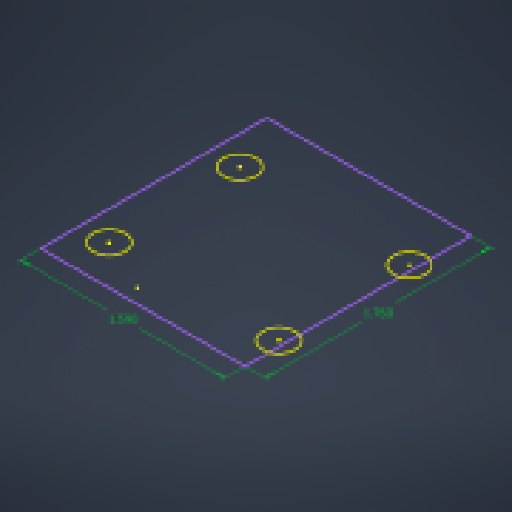
# Autodesk Inventor part: WheelBracketConnector
Saved by Autodesk Inventor 2027 (Build 310192000, 192)
## iProperties
Created: 2026-07-09
Part Number: WheelBracketConnector
Material: Generic
Document SubType Name: Modeling
Designer: belcz
Density: 1 g/cm^3
Appearance: Default
Author: belcz
Autodesk Inventor part; units mm, degrees
ref_plane "YZ Plane" through (0, 0, 0) normal (1, 0, 0) x (0, 1, 0)
ref_plane "XZ Plane" through (0, 0, 0) normal (0, 1, 0) x (-1, 0, 0)
ref_plane "XY Plane" through (0, 0, 0) normal (0, 0, 1) x (1, 0, 0)
sketch "Sketch1" plane through (0, 0, 0) normal (0, 1, 0) x (-1, 0, 0)
  circle A0 centre (10.7243, -30.9952) radius 3.175 projected
  circle A1 centre (10.7243, -5.1761) radius 3.175 projected
  circle A2 centre (-22.8037, -5.1761) radius 3.175 projected
  circle A3 centre (-22.8037, -30.9952) radius 3.175 projected
  line L0 (16.4239, -38.285) -> (-28.2801, -38.285)
  line L1 (-28.2801, -38.285) -> (-28.2801, 2.101)
  line L2 (-28.2801, 2.101) -> (16.4239, 2.101)
  line L3 (16.4239, 2.101) -> (16.4239, -38.285)
  circle A4 centre (-22.8037, -30.9952) radius 3.683
  circle A5 centre (-22.8037, -5.1761) radius 3.683
  circle A6 centre (10.7243, -5.1761) radius 3.683
  circle A7 centre (10.7243, -30.9952) radius 3.683
  line L4 (-28.2801, 2.101) -> (16.4239, 2.101)
  line L5 (16.4239, 2.101) -> (16.4239, -38.285)
  line L6 (16.4239, -38.285) -> (-28.2801, -38.285)
  line L7 (-28.2801, -38.285) -> (-28.2801, 2.101)
  circle A8 centre (10.7243, -5.1761) radius 3.175
  circle A9 centre (10.7243, -30.9952) radius 3.175
  circle A10 centre (-22.8037, -30.9952) radius 3.175
  circle A11 centre (-22.8037, -5.1761) radius 3.175
  point P0 (0, 0)
  dimension "d0" = 44.704
  dimension "d1" = 40.386
  dimension "d2" = 7.2898
  dimension "d3" = 7.2771
  dimension "d4" = 7.366
  dimension "d5" = 7.366
  dimension "d6" = 7.366
  dimension "d7" = 7.366
  constraints: 16 end point, 8 centre point, 8 coincident, 4 concentric, 4 parallel, 2 horizontal, 2 perpendicular
  measures "d0" distance of L1.end L2.end
  measures "d1" distance of L0.end L1.end
  measures "d2" distance from line of L0 A3.centre
  measures "d3" distance from line of L2 A2.centre
  measures "d4" diameter of A4
  measures "d5" diameter of A5
  measures "d6" diameter of A6
  measures "d7" diameter of A7
extrude "Extrusion1" add sketch "Sketch1" along normal blind 4.826 contours A4 | A5 | A6 | A7
sketch "Sketch2" plane through (-10.7243, 0, -30.9952) normal (0, -1, 0) x (1, 0, 0)
  line L0 (39.0044, 33.0962) -> (-5.6996, 33.0962) projected
  line L1 (39.0044, -7.2898) -> (39.0044, 33.0962) projected
  line L2 (-5.6996, -7.2898) -> (39.0044, -7.2898) projected
  line L3 (-5.6996, 33.0962) -> (-5.6996, -7.2898) projected
  line L4 (39.0044, 33.0962) -> (-5.6996, 33.0962)
  line L5 (-5.6996, 33.0962) -> (-5.6996, -7.2898)
  line L6 (-5.6996, -7.2898) -> (39.0044, -7.2898)
  line L7 (39.0044, -7.2898) -> (39.0044, 33.0962)
  circle A0 centre (33.528, 0) radius 3.175 projected
  circle A1 centre (0, 0) radius 3.175 projected
  circle A2 centre (0, 25.8191) radius 3.175 projected
  circle A3 centre (33.528, 25.8191) radius 3.175 projected
  circle A4 centre (33.528, 0) radius 3.175
  circle A5 centre (0, 0) radius 3.175
  circle A6 centre (0, 25.8191) radius 3.175
  circle A7 centre (33.528, 25.8191) radius 3.175
  point P0 (10.7243, 30.9952)
  constraints: 8 end point, 4 centre point, 4 coincident, 4 concentric, 2 parallel, 1 horizontal, 1 perpendicular
extrude "Extrusion2" add sketch "Sketch2" against normal blind 3.2131
fillet "Fillet1" radius 3.175 4 edges at (-16.4239, 1.6065, 2.101) (28.2801, 1.6065, 2.101) (28.2801, 1.6065, -38.285) (-16.4239, 1.6065, -38.285)
thread "Thread1" size "1/4-20 UNC" class "2B" standard "ANSI Unified Screw Threads" full length
thread "Thread2" size "1/4-20 UNC" class "2B" standard "ANSI Unified Screw Threads" full length
thread "Thread3" size "1/4-20 UNC" class "2B" standard "ANSI Unified Screw Threads" full length
thread "Thread4" size "1/4-20 UNC" class "2B" standard "ANSI Unified Screw Threads" full length
body "Solid1"
